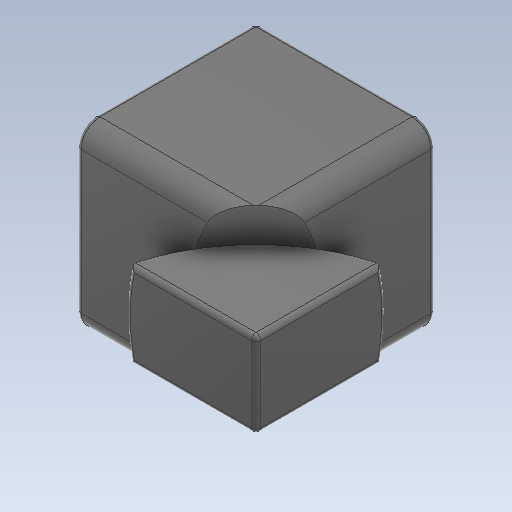
# Autodesk Inventor part: middle-piece
Saved by Autodesk Inventor 2020 (Build 240168000, 168)
## iProperties
Created: 2019-10-07
Part Number: middle-piece
Material: Generic
Document SubType Name: Modeling
Designer: eduso287260
Density: 1 g/cm^3
Appearance: Default
Author: eduso287260
Autodesk Inventor part; units mm, degrees
ref_plane "YZ Plane" through (0, 0, 0) normal (1, 0, 0) x (0, 1, 0)
ref_plane "XZ Plane" through (0, 0, 0) normal (0, 1, 0) x (-1, 0, 0)
ref_plane "XY Plane" through (0, 0, 0) normal (0, 0, 1) x (1, 0, 0)
sketch "Sketch2" plane through (0, 0, 0) normal (0, 1, 0) x (-1, 0, 0)
  circle A0 centre (0, 0) radius 19
  line L0 (9.5, -9.5) -> (28.5, -9.5)
  line L1 (28.5, -9.5) -> (28.5, -28.5)
  line L2 (28.5, -28.5) -> (9.5, -28.5)
  line L3 (9.5, -28.5) -> (9.5, -9.5)
  line L4 (48.3678, 0) -> (-30.228, 0)
  line L5 (0, -38.6327) -> (0, 32.2963) projected
  line L6 (20.1631, 0) -> (-22.04, 0)
  line L7 (18.4594, -4.5) -> (0, -4.5)
  line L8 (4.5, 0) -> (4.5, -18.4594)
  line L9 (18.4594, -4.5) -> (20.661, -4.5)
  line L10 (20.661, -4.5) -> (20.661, 22.1636)
  line L11 (20.661, 22.1636) -> (-21.4163, 22.1636)
  line L12 (-21.4163, 22.1636) -> (-21.4163, -22.8512)
  line L13 (-21.4163, -22.8512) -> (4.5, -22.8512)
  line L14 (4.5, -22.8512) -> (4.5, -18.4594)
  point P0 (0, -19)
  point P1 (19, 0)
  point P2 (4.5, -4.5)
  dimension "d0" = 38
  dimension "d1" = 19
  dimension "d2" = 19
  dimension "d3" = 9.5
  dimension "d4" = 9.5
  dimension "d8" = 4.5
  dimension "d9" = 4.5
  constraints: 28 end point, 7 perpendicular, 4 point on line, 2 horizontal, 2 parallel, 2 point on circle, 1 centre point, 1 coincident, 1 collinear
  measures "d0" diameter of A0
  measures "d1" distance of L1.end L2.end
  measures "d2" distance of L0.end L1.end
  measures "d3" distance between parallel lines of L0 L4
  measures "d4" distance between parallel lines of L3 L5
  measures "d8" distance between parallel lines of L4 L7
  measures "d9" distance between parallel lines of L5 L8
extrude "Extrusion1" add sketch "Sketch2" along normal mid plane 19 contours L0 L1 L2 L3 A0 | A0 L3 L0
revolve "Revolution1" cut sketch "Sketch2" angle 110 mid plane about axis through (-48.3678, 0, 0) along (1, 0, 0) contours L7 L8 L4 A0 | A0 L0 L3 L8 L7 | A0 L3 L0 | L8 A0 L5 L7 | L7 L5 L4 L8
sketch "Sketch3" plane through (0, 0, 0) normal (0, 1, 0) x (-1, 0, 0)
  circle A0 centre (0, 0) radius 19
  line L0 (-13.1034, -13.7586) -> (13.1034, 13.7586)
  dimension "d10" = 38
  constraints: 2 end point, 2 point on circle, 1 centre point, 1 coincident, 1 midpoint
  measures "d10" diameter of A0
revolve "Revolution2" add sketch "Sketch3" angle 360 about axis through (13.1034, 0, -13.7586) along (-0.6896552, 0, 0.7241379) separate body picked at (4.8459, -4.0778) contours A0 L0
extrude "Extrusion2" cut sketch "Sketch2" along normal mid plane 55.75 contours L7 L8 L4 A0 | A0 L4 L10 L9 | L4 L5 A0 | A0 L5 L11 L10 L4 | L8 A0 L5 L7 | L7 L5 L4 L8 | L5 L4 A0 | A0 L4 L12 L11 L5 | L5 A0 L4 | L14 L13 L5 A0 | A0 L5 L13 L12 L4 bodies 2
sketch "Sketch4" plane through (0, 0, 0) normal (0, 1, 0) x (-1, 0, 0)
  line L0 (22.2405, 22.0402) -> (-22.2405, 22.0402)
  line L1 (-22.2405, 22.0402) -> (-22.2405, -22.0402)
  line L2 (-22.2405, -22.0402) -> (22.2405, -22.0402)
  line L3 (22.2405, -22.0402) -> (22.2405, 22.0402)
  line L4 (22.2405, 22.0402) -> (-22.2405, -22.0402) construction
  line L5 (-22.2405, 22.0402) -> (22.2405, -22.0402) construction
  point P0 (0, 0)
  constraints: 12 end point, 2 midpoint, 2 parallel, 1 horizontal, 1 perpendicular
extrude "Extrusion3" cut sketch "Sketch4" along normal mid plane 9 keep common part bodies 2
fillet "Fillet1" radius 2 4 edges at (-20.9675, 9.5, -9.5) (-9.5, 9.5, -20.9675) (-20.9675, -9.5, -9.5) (-9.5, -9.5, -20.9675)
fillet "Fillet2" radius 0.5 11 edges at (-28.5, 0, -28.5) (-28.5, -8.9142, -10.0858) (-28.5, -9.5, -20) (-28.5, 8.9142, -10.0858) (-28.5, 9.5, -20) (-28.5, 0, -9.5) (-10.0858, 8.9142, -28.5) (-9.5, 0, -28.5) (-10.0858, -8.9142, -28.5) (-20, -9.5, -28.5) (-20, 9.5, -28.5)
combine bodies "Combine1" operation type add bodies to combine 1 2
fillet "Fillet3" radius 0.5 7 edges at (-4.5, 4.5, -11.2013) (-11.2013, 4.5, -4.5) (-11.2013, -4.5, -4.5) (-4.5, -4.5, -11.2013) (-4.5, 0, -18.4594) (-18.4594, 0, -4.5) (-4.5, 0, -4.5)
sketch "Sketch5" plane through (-28.5, -9, -28) normal (-1, 0, 0) x (0, 0, 1)
  line L0 (1.5, 0.5) -> (16.5, 0.5)
  line L1 (17.5, 1.5) -> (17.5, 16.5)
  line L2 (16.5, 17.5) -> (1.5, 17.5)
  line L3 (0.5, 16.5) -> (0.5, 1.5)
  line L4 (0.5, 0.5) -> (17.5, 17.5) construction
  line L5 (17.5, 0.5) -> (0.5, 17.5) construction
  line L6 (-0.5, 18) -> (-0.5, 0) projected
  line L7 (16.5, 18.5) -> (0, 18.5) projected
  line L8 (1.5, 1.5) -> (16.5, 1.5)
  line L9 (16.5, 1.5) -> (16.5, 16.5)
  line L10 (16.5, 16.5) -> (1.5, 16.5)
  line L11 (1.5, 16.5) -> (1.5, 1.5)
  line L12 (1.5, 1.5) -> (16.5, 16.5) construction
  line L13 (16.5, 1.5) -> (1.5, 16.5) construction
  arc A0 (1.5, 17.5) -> (0.5, 16.5) centre (1.5, 16.5) ccw
  arc A1 (0.5, 1.5) -> (1.5, 0.5) centre (1.5, 1.5) ccw
  arc A2 (16.5, 0.5) -> (17.5, 1.5) centre (16.5, 1.5) ccw
  arc A3 (17.5, 16.5) -> (16.5, 17.5) centre (16.5, 16.5) ccw
  point P0 (28, 9)
  point P1 (9, 9)
  dimension "d19" = 17
  dimension "d20" = 17
  dimension "d21" = 1
  dimension "d22" = 1
  dimension "d23" = 15
  dimension "d24" = 15
  dimension "d25" = 1
  constraints: 24 end point, 8 point on circle, 8 point on line, 8 tangent, 4 centre point, 4 midpoint, 4 parallel, 3 equal radius, 2 horizontal, 2 perpendicular
  measures "d19" distance of L5.end L4.end
  measures "d20" distance of L4.end L5.start
  measures "d21" distance between parallel lines of L3 L6
  measures "d22" distance between parallel lines of L7 L2
  measures "d23" distance of L10.end L9.end
  measures "d24" distance of L9.end L8.end
  measures "d25" radius of A0
extrude "Extrusion4" cut sketch "Sketch5" against normal blind 2 contours L11 L10 L9 L8 bodies 1
extrude "Extrusion5" cut sketch "Sketch5" against normal blind 1 bodies 1
fillet "Fillet4" radius 0.25 8 edges at (-28.5, 8.2071, -10.7929) (-28.5, 0, -10.5) (-28.5, -8.2071, -10.7929) (-28.5, -8.5, -19) (-28.5, -8.2071, -27.2071) (-28.5, 0, -27.5) (-28.5, 8.2071, -27.2071) (-28.5, 8.5, -19)
sketch "Sketch6" plane through (-11.5, 9, -28.5) normal (0, 0, -1) x (-1, 0, 0)
  line L0 (0, -17.5) -> (15, -17.5)
  line L1 (16, -16.5) -> (16, -1.5)
  line L2 (15, -0.5) -> (0, -0.5)
  line L3 (-1, -1.5) -> (-1, -16.5)
  line L4 (-1, -17.5) -> (16, -0.5) construction
  line L5 (16, -17.5) -> (-1, -0.5) construction
  line L6 (17, -18) -> (17, 0) projected
  line L7 (0, -18.5) -> (16.5, -18.5) projected
  line L8 (0, -16.5) -> (15, -16.5)
  line L9 (15, -16.5) -> (15, -1.5)
  line L10 (15, -1.5) -> (0, -1.5)
  line L11 (0, -1.5) -> (0, -16.5)
  line L12 (0, -16.5) -> (15, -1.5) construction
  line L13 (15, -16.5) -> (0, -1.5) construction
  arc A0 (0, -0.5) -> (-1, -1.5) centre (0, -1.5) ccw
  arc A1 (-1, -16.5) -> (0, -17.5) centre (0, -16.5) ccw
  arc A2 (15, -17.5) -> (16, -16.5) centre (15, -16.5) ccw
  arc A3 (16, -1.5) -> (15, -0.5) centre (15, -1.5) ccw
  point P0 (-11.5, -9)
  point P1 (7.5, -9)
  dimension "d31" = 17
  dimension "d32" = 17
  dimension "d33" = 1
  dimension "d34" = 1
  dimension "d35" = 15
  dimension "d36" = 15
  dimension "d37" = 1
  constraints: 24 end point, 8 point on circle, 8 point on line, 8 tangent, 4 centre point, 4 midpoint, 4 parallel, 3 equal radius, 2 horizontal, 2 perpendicular
  measures "d31" distance of L5.end L4.end
  measures "d32" distance of L4.end L5.start
  measures "d33" distance between parallel lines of L6 L1
  measures "d34" distance between parallel lines of L7 L0
  measures "d35" distance of L10.end L9.end
  measures "d36" distance of L9.end L8.end
  measures "d37" radius of A0
extrude "Extrusion6" cut sketch "Sketch6" against normal blind 2 contours L11 L10 L9 L8 bodies 1
extrude "Extrusion7" cut sketch "Sketch6" against normal blind 1 bodies 1
body "Solid1"
